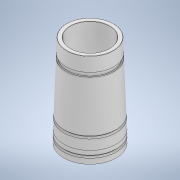
# Autodesk Inventor part: Part1
Saved by Autodesk Inventor 2020 (Build 240168000, 168)
## iProperties
Created: 2020-03-27
Part Number: Part1
Material: Aluminum 2014-T6
Document SubType Name: Modeling
Designer: User
Density: 2.78927 g/cm^3
Appearance: Satin
Author: User
Autodesk Inventor part; units mm, degrees
ref_plane "YZ Plane" through (0, 0, 0) normal (1, 0, 0) x (0, 1, 0)
ref_plane "XZ Plane" through (0, 0, 0) normal (0, 1, 0) x (-1, 0, 0)
ref_plane "XY Plane" through (0, 0, 0) normal (0, 0, 1) x (1, 0, 0)
sketch "Sketch1" plane through (0, 0, 0) normal (1, 0, 0) x (0, 1, 0)
  line L0 (-20, 0) -> (70, 0)
  line L1 (0, 0) -> (0, -20)
  line L2 (0, -20) -> (9.148, -20)
  line L3 (9.148, -20) -> (70, -17.875)
  line L4 (70, 0) -> (70, -17.875)
  line L5 (3, -10) -> (3, -17)
  line L6 (7.8773, 0) -> (3, -10)
  line L7 (7.8773, 0) -> (19.0033, 0) construction
  line L8 (10, 0) -> (10, -16.9852)
  line L9 (9.5775, -17) -> (70, -14.89)
  line L10 (3, -17) -> (9.5775, -17)
  line L11 (70, -17.875) -> (69.8959, -14.8936)
  line L12 (6.0374, -20) -> (4.9651, -19)
  line L13 (4.9651, -19) -> (4.0326, -20)
  line L14 (4.9651, -19) -> (5, -20)
  line L15 (17.532, -19.7072) -> (17.4971, -18.7078)
  line L16 (17.4971, -18.7078) -> (18.5314, -19.6723)
  line L17 (17.4971, -18.7078) -> (16.5326, -19.7421)
  line L18 (59.5059, -18.2415) -> (56.5082, -18.3461)
  line L19 (56.5082, -18.3461) -> (56.4733, -17.3468)
  line L20 (56.4733, -17.3468) -> (59.4729, -17.2944)
  line L21 (59.4729, -17.2944) -> (59.5059, -18.2415)
  line L22 (0.5, 0) -> (0.5, -1)
  line L23 (0, -1.5) -> (0.5, -1)
  line L24 (0.5, -1) -> (5, -1)
  line L25 (5, -1) -> (5.5774, 0)
  line L26 (0.25, -1.25) -> (4, -1.25)
  line L27 (4, -1.25) -> (4, 0)
  point P0 (4, -1)
  dimension "d0" = 90
  dimension "d1" = 20
  dimension "d4" = 70
  dimension "d5" = 3
  dimension "d6" = 116
  dimension "d8" = 10
  dimension "d10" = 7
  dimension "d14" = 17.875
  dimension "d15" = 14.89
  dimension "d16" = 88
  dimension "d17" = 88
  dimension "d18" = 90
  dimension "d22" = 5
  dimension "d23" = 1
  dimension "d24" = 1
  dimension "d25" = 52.5
  dimension "d26" = 3
  dimension "d27" = 1
  dimension "d28" = 13.5
  dimension "d29" = 0.5
  dimension "d33" = 4.5
  dimension "d34" = 60
  dimension "d35" = 1.25
  dimension "d36" = 4
  constraints: 56 end point, 16 point on line, 6 horizontal, 5 perpendicular, 5 vertical, 1 equal length, 1 midpoint, 1 parallel, 2 other
  measures "d0" distance of L0.start L0.end
  measures "d1" distance of L1.start L1.end
  measures "d4" distance between parallel lines of L1 L4
  measures "d5" distance between parallel lines of L1 L5
  measures "d6" angle of L6 L7
  measures "d8" distance from line of L5.start L0
  measures "d10" distance between parallel lines of L5 L8
  measures "d14" distance of L3.end L0.end
  measures "d15" distance of L9.end L0.end
  measures "d16" angle of L4 L3
  measures "d17" angle of L4 L9
  measures "d18" angle of L13 L12
  measures "d22" distance from line of L1 L14.end
  measures "d23" vertical distance of L12.end L14.end
  measures "d24" distance of L15.start L15.end
  measures "d25" distance between parallel lines of L11 L15
  measures "d26" distance of L19.end L20.end
  measures "d27" distance of L18.end L19.end
  measures "d28" distance between parallel lines of L19 L11
  measures "d29" distance from line of L1 L22.end
  measures "d33" distance of L22.end L24.end
  measures "d34" angle of L0 L25
  measures "d35" distance between parallel lines of L0 L26
  measures "d36" distance from line of L1 L26.end
revolve "Revolution1" add sketch "Sketch1" angle 360 about axis through (0, -20, 0) along (0, 1, 0) contours L23 L26 L27 L24 L25 L0 L6 L5 L10 L9 L11 L3 L21 L20 L19 L16 L17 L2 L12 L13 L1
fillet "Fillet1" radius 0.2 2 edges at (0, 70, 17.875) (0, 69.8959, 14.8936)
thread "Thread2" size "M2.5x0.45" class "6H" standard "ANSI Metric M Profile" length 3.5
body "Solid1"
